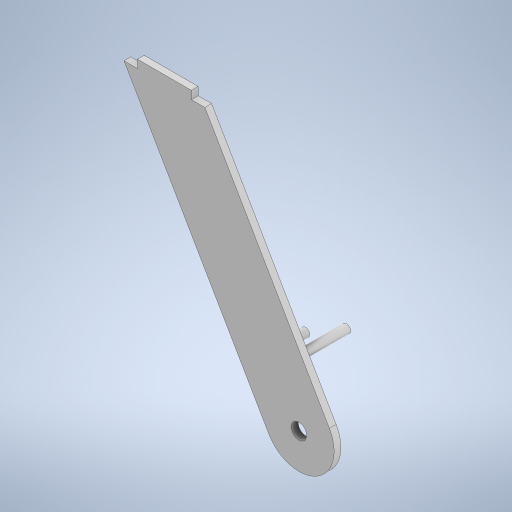
# Autodesk Inventor part: bacak
Saved by Autodesk Inventor 2023.2 (Build 272271000, 271)
## iProperties
Created: 2022-11-26
Part Number: bacak
Material: Generic
Document SubType Name: Modeling
Designer: omrfrkmll
Density: 1 g/cm^3
Appearance: Default
Author: omrfrkmll
Autodesk Inventor part; units mm, degrees
ref_plane "YZ Plane" through (0, 0, 0) normal (1, 0, 0) x (0, 1, 0)
ref_plane "XZ Plane" through (0, 0, 0) normal (0, 1, 0) x (-1, 0, 0)
ref_plane "XY Plane" through (0, 0, 0) normal (0, 0, 1) x (1, 0, 0)
sketch "Sketch1" plane through (0, 0, 0) normal (0, 0, 1) x (1, 0, 0)
  line L0 (-16.8629, 0) -> (19.5362, 0)
  line L1 (0, 12.2153) -> (0, -13.8193)
  line L2 (-10, 1.5) -> (10, 1.5)
  line L3 (10, 1.5) -> (10, -1.5)
  line L4 (10, -1.5) -> (-10, -1.5)
  line L5 (-10, -1.5) -> (-10, 1.5)
  point P0 (0, 0)
  point P1 (0, -1.5)
  point P2 (0, 1.5)
  dimension "d0" = 3
  dimension "d1" = 20
  constraints: 12 end point, 3 horizontal, 2 parallel, 2 vertical, 1 perpendicular, 3 other
  measures "d0" distance between parallel lines of L4 L2
  measures "d1" distance between parallel lines of L5 L3
sketch "Sketch3" plane through (0, 0, 0) normal (0, 0, 1) x (1, 0, 0)
  line L0 (0, 4.1951) -> (0, -4.771)
  line L1 (-15, -1.5) -> (15, -1.5)
  line L2 (15, -1.5) -> (61.188, -81.5)
  line L3 (-15, -1.5) -> (38.688, -94.4904)
  line L4 (-13.3896, 0) -> (12.5963, 0)
  line L5 (-10, -1.5) -> (10, -1.5) projected
  line L6 (0, -1.5) -> (34.9904, -62.1052)
  arc A0 (38.688, -94.4904) -> (61.188, -81.5) centre (49.938, -87.9952) ccw
  line L7 (-16.4414, -1.5) -> (20.4341, -1.5)
  point P0 (0, 0)
  point P1 (0, -0.2879)
  dimension "d20" = 30
  dimension "d22" = 60
  dimension "d23" = 80
  dimension "d24" = 3
  constraints: 14 end point, 3 horizontal, 3 point on line, 2 midpoint, 2 parallel, 2 point on circle, 2 vertical, 1 centre point, 1 symmetric about line, 1 tangent
  measures "d20" distance of L1.start L1.end
  measures "d22" angle of L2 L1
  measures "d23" distance from line of L1 L2.end
  measures "d24" diameter of L1 L4
extrude "Extrusion1" add sketch "Sketch3" along normal mid plane 2.5
sketch "Sketch5" plane through (0, 0, 1.25) normal (0, 0, 1) x (1, 0, 0)
  arc A0 (38.688, -94.4904) -> (61.188, -81.5) centre (49.938, -87.9952) ccw projected
  point P0 (0, 0)
  point P1 (38.391, -42.0144)
  constraints: 1 coincident
hole "Hole1" at (49.938, -87.9952, 1.25) direction (0, 0, -1) diameter 5.6 end through all
sketch "Sketch6" plane through (0, 0, 1.25) normal (0, 0, 1) x (1, 0, 0)
  line L0 (21.1799, -20.6847) -> (35.9337, -46.239)
  line L1 (4.4808, -26.761) -> (20.9112, -55.2193)
  line L2 (61.188, -81.5) -> (15, -1.5) projected
  line L3 (32.3354, -75.0065) -> (47.4908, -66.2565)
  circle A0 centre (47.4908, -66.2565) radius 1.55
  circle A1 centre (32.3354, -75.0065) radius 1.55
  circle A2 centre (49.938, -87.9952) radius 2.8 projected
  line L4 (49.938, -87.9952) -> (10.4204, -19.5487)
  line L5 (47.4908, -66.2565) -> (49.938, -87.9952)
  point P0 (0, 0)
  point P1 (38.391, -42.0144)
  dimension "d25" = 17.5
  dimension "d26" = 3.1
  dimension "d27" = 3.1
  dimension "d32" = 21.876
  constraints: 10 end point, 2 centre point, 2 coincident, 2 parallel, 2 point on line, 1 perpendicular, 2 other
  measures "d25" distance between parallel lines of L1 L0
  measures "d26" diameter of A0
  measures "d27" diameter of A1
  measures "d32" distance of L4.start L5.start
extrude "Extrusion3" add sketch "Sketch6" against normal blind 20 contours A0 L5 L3 | L3 L5 A0 | A1
extrude "Extrusion4" add sketch "Sketch1" along normal mid plane 2.5
body "Solid1"
